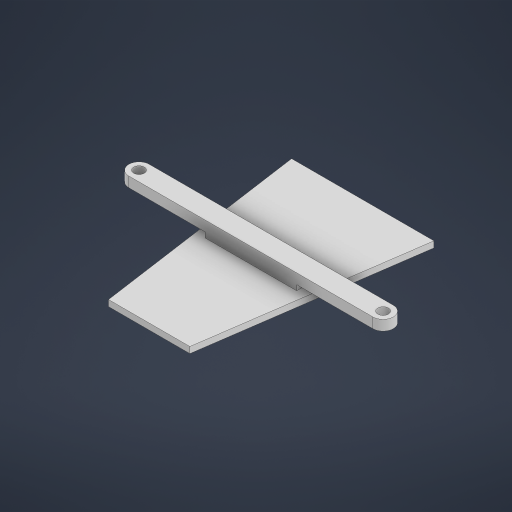
# Autodesk Inventor part: karoserie2
Saved by Autodesk Inventor 2023 (Build 270158000, 158)
## iProperties
Created: 2024-04-15
Part Number: karoserie2
Material: Generic
Document SubType Name: Modeling
Designer: Matooš
Density: 1 g/cm^3
Appearance: Default
Author: Matooš
Autodesk Inventor part; units mm, degrees
ref_plane "YZ Plane" through (0, 0, 0) normal (1, 0, 0) x (0, 1, 0)
ref_plane "XZ Plane" through (0, 0, 0) normal (0, 1, 0) x (-1, 0, 0)
ref_plane "XY Plane" through (0, 0, 0) normal (0, 0, 1) x (1, 0, 0)
sketch "Sketch1" plane through (0, 0, 0) normal (0, 1, 0) x (-1, 0, 0)
  line L0 (0, -66) -> (0, 81) projected
  line L1 (-49, 0) -> (49, 0) projected
  line L2 (-35, -45) -> (35, -45)
  line L3 (20, 60) -> (-20, 60)
  line L4 (-20, 60) -> (-35, -45)
  line L5 (35, -45) -> (20, 60)
  point P0 (0, 0)
  dimension "d0" = 70
  dimension "d1" = 105
  dimension "d3" = 40
  dimension "d6" = 45
  constraints: 8 end point, 1 horizontal, 1 parallel, 1 other
  measures "d0" distance of L2.start L2.end
  measures "d1" distance between parallel lines of L3 L2
  measures "d3" distance of L3.start L3.end
  measures "d6" distance between parallel lines of L1 L2
extrude "Extrusion1" add sketch "Sketch1" along normal blind 3
sketch "Sketch2" plane through (0, 0, 0) normal (0, 0, 1) x (1, 0, 0)
  line L0 (-91, 0) -> (91, 0) projected
  line L1 (0, 12.72) -> (0, -2.12) projected
  line L2 (35, 3) -> (-35, 3) projected
  line L3 (22.5, 3) -> (-22.5, 3)
  line L4 (-22.5, 3) -> (-22.5, 5.6)
  line L5 (22.5, 5.6) -> (22.5, 3)
  line L6 (22.5, 5.6) -> (65, 5.6)
  line L7 (65, 5.6) -> (65, 10.6)
  line L8 (65, 10.6) -> (-65, 10.6)
  line L9 (-65, 10.6) -> (-65, 5.6)
  line L10 (-65, 5.6) -> (-22.5, 5.6)
  line L11 (-35, 0) -> (-35, 3) projected
  line L12 (35, 0) -> (35, 3) projected
  point P0 (0, 0)
  point P1 (-22.5, 3)
  point P2 (22.5, 3)
  dimension "d8" = 2.6
  dimension "d9" = 130
  dimension "d10" = 5
  dimension "d11" = 2.6
  dimension "d22" = 45
  constraints: 16 end point, 5 perpendicular, 2 horizontal, 1 collinear, 1 parallel, 2 other
  measures "d8" distance of L5.start L3.start
  measures "d9" distance of L7.end L8.end
  measures "d10" distance between parallel lines of L8 L6
  measures "d11" distance of L3.end L4.end
  measures "d22" distance between parallel lines of L5 L4
extrude "Extrusion2" add sketch "Sketch2" along normal blind 10 contours L2 L4 L10 L9 L8 L1 | L1 L8 L7 L6 L5 L2
fillet "Fillet1" radius 5 4 edges at (65, 8.1, 0) (65, 8.1, 10) (-65, 8.1, 0) (-65, 8.1, 10)
sketch "Sketch3" plane through (-60, 10.6, 0) normal (0, 1, 0) x (1, 0, 0)
  arc A0 (0, 0) -> (0, -10) centre (0, -5) ccw projected
  arc A1 (120, -10) -> (120, 0) centre (120, -5) ccw projected
  point P0 (60, 0)
  constraints: 2 coincident
hole "Hole1" at (60, 10.6, 5) at (-60, 10.6, 5) direction (0, -1, 0) diameter 5.2 end through all
body "Solid1"
